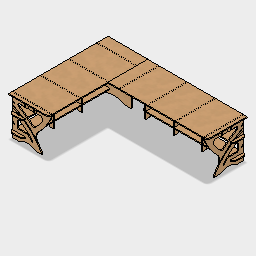
Corner bench (Autodesk Fusion 360 design; units mm, degrees)
Autodesk Fusion 360 part; units mm, degrees
note: some values were not read from the file. Set by a fixed rule: which sketch regions a step uses.
(part 1 of 2)
sketch "Inner end leg" plane through (0, 0, 0) normal (0, 0, 1) x (1, 0, 0)
  circle A0 centre (-454.5584, 695.833) radius 3.175
  line L0 (-307.4416, 743.458) -> (-289.4584, 743.458) construction
  line L1 (-454.5584, 692.658) -> (-472.5416, 692.658)
  line L2 (-472.5416, 692.658) -> (-472.5416, 749.6387)
  line L3 (-307.4416, 692.658) -> (-307.4416, 749.6387)
  circle A1 centre (-123.825, 133.858) radius 3.175
  line L4 (-454.5584, 749.6387) -> (-454.5584, 692.658)
  circle A2 centre (-307.4416, 695.833) radius 3.175
  circle A3 centre (-123.825, 115.8748) radius 3.175
  line L5 (-472.5416, 743.458) -> (-454.5584, 743.458) construction
  circle A4 centre (-472.5416, 695.833) radius 3.175
  circle A5 centre (-289.4584, 695.833) radius 3.175
  line L6 (-289.4584, 749.6387) -> (-289.4584, 692.658)
  line L7 (-289.4584, 692.658) -> (-307.4416, 692.658)
  line L8 (0, 288.3803) -> (-40.4112, 247.9691)
  line L9 (-31.4309, 238.9888) -> (-5.4201, 264.9997)
  arc A6 (-40.4112, 584.3498) -> (-31.4309, 575.3695) centre (-35.921, 579.8596) ccw
  arc A7 (-40.4112, 247.9691) -> (-31.4309, 238.9888) centre (-35.921, 243.479) ccw
  line L10 (0, 133.858) -> (-127, 133.858)
  line L11 (0, 429.6664) -> (-127, 429.6664) construction
  line L12 (-127, 115.8748) -> (0, 115.8748)
  line L13 (0, 124.8664) -> (-127, 124.8664) construction
  circle A8 centre (-123.825, 420.6748) radius 3.175
  line L14 (-127, 133.858) -> (-127, 115.8748)
  circle A9 centre (-123.825, 438.658) radius 3.175
  line L15 (0, 624.7609) -> (-40.4112, 584.3498)
  line L16 (-35.921, 579.8596) -> (0, 615.7807) construction
  line L17 (0, 438.658) -> (-127, 438.658)
  line L18 (0, 279.4) -> (-35.921, 243.479) construction
  line L19 (-31.4309, 575.3695) -> (-5.4201, 601.3803)
  line L20 (-127, 420.6748) -> (0, 420.6748)
  line L21 (-127, 438.658) -> (-127, 420.6748)
  line L22 (-660.4, 749.6387) -> (-660.4, 0)
  line L23 (-112.121, 629.158) -> (-558.8, 629.158)
  line L24 (-584.2, 603.758) -> (-584.2, 527.558)
  line L25 (-558.8, 502.158) -> (-112.121, 502.158)
  line L26 (-86.721, 527.558) -> (-86.721, 603.758)
  line L27 (-112.121, 357.1748) -> (-558.8, 357.1748)
  line L28 (-584.2, 331.7748) -> (-584.2, 222.758)
  line L29 (-558.8, 197.358) -> (-112.121, 197.358)
  line L30 (-86.721, 222.758) -> (-86.721, 331.7748)
  arc A10 (-86.721, 603.758) -> (-112.121, 629.158) centre (-112.121, 603.758) ccw
  arc A11 (-558.8, 629.158) -> (-584.2, 603.758) centre (-558.8, 603.758) ccw
  arc A12 (-584.2, 527.558) -> (-558.8, 502.158) centre (-558.8, 527.558) ccw
  arc A13 (-112.121, 502.158) -> (-86.721, 527.558) centre (-112.121, 527.558) ccw
  arc A14 (-86.721, 331.7748) -> (-112.121, 357.1748) centre (-112.121, 331.7748) ccw
  arc A15 (-558.8, 357.1748) -> (-584.2, 331.7748) centre (-558.8, 331.7748) ccw
  arc A16 (-584.2, 222.758) -> (-558.8, 197.358) centre (-558.8, 222.758) ccw
  arc A17 (-112.121, 197.358) -> (-86.721, 222.758) centre (-112.121, 222.758) ccw
  arc A18 (-101.6, 0) -> (-558.8, 0) centre (-330.2, -488.95) ccw
  line L31 (-660.4, 0) -> (-558.8, 0)
  line L32 (-101.6, 0) -> (0, 0)
  line L33 (0, 749.6387) -> (-289.4584, 749.6387)
  line L34 (-307.4416, 749.6387) -> (-454.5584, 749.6387)
  line L35 (-472.5416, 749.6387) -> (-660.4, 749.6387)
  line L36 (0, 624.7609) -> (0, 749.6387)
  line L37 (0, 599.1353) -> (0, 624.7609) construction
  line L38 (0, 438.658) -> (0, 599.1353)
  line L39 (0, 288.3803) -> (0, 420.6748)
  line L40 (0, 0) -> (0, 115.8748)
  line L41 (0, 400.0363) -> (0, 288.3803) construction
  line L42 (0, 133.858) -> (0, 262.7546)
  arc A19 (0, 599.1353) -> (-5.4201, 601.3803) centre (-3.175, 599.1353) ccw
  arc A20 (0, 262.7546) -> (-5.4201, 264.9997) centre (-3.175, 262.7546) ccw
  line L43 (0, 420.6748) -> (0, 438.658) construction
  line L44 (0, 115.8748) -> (0, 133.858) construction
  line L45 (0, 288.3803) -> (0, 262.7546) construction
  line L46 (-101.6, 0) -> (-558.8, 0) construction
  line L47 (-330.2, 0) -> (-330.2, 50.8) construction
  point P0 (0, 429.6664)
  point P1 (-298.45, 743.458)
  point P2 (-381, 749.6387)
  point P3 (-463.55, 743.458)
  point P4 (-558.8, 0)
  point P5 (-101.6, 0)
  dimension "d1011" = 50.8
  dimension "d1015" = 50.8
  dimension "d1017" = 17.9832
  dimension "d1019" = 6.35
  dimension "d1020" = 6.35
  dimension "d1021" = 17.9832
  dimension "d1023" = 6.35
  dimension "d1024" = 6.35
  dimension "d1025" = 8.9916
  dimension "d1026" = 8.9916
  dimension "d1034" = 50.8
  dimension "d1036" = 50.8
  dimension "d1037" = 6.35
  dimension "d1038" = 6.35
  dimension "d1039" = 6.35
  dimension "d1040" = 6.35
  dimension "d1042" = 82.55
  dimension "d1043" = 82.55
  dimension "d1062" = 133.858
  dimension "d1063" = 438.658
  dimension "d1103" = 63.5
  dimension "d1104" = 63.5
  dimension "d1105" = 50.8
  dimension "d1106" = 76.2
  dimension "d1107" = 76.2
  dimension "d1108" = 50.8
  dimension "d1109" = 63.5
  dimension "d1110" = 63.5
  dimension "d1114" = 25.4
  dimension "d1115" = 25.4
  dimension "d1250" = 101.6
  dimension "d2612" = 3.175
  dimension "d2613" = 3.175
  dimension "d2750" = 6.35
  dimension "d2751" = 6.35
  dimension "d2961" = 45
  dimension "d2962" = 127
  dimension "d2964" = 101.6
  dimension "d2965" = 127
  dimension "d2966" = 45
  dimension "d2967" = 279.4
  dimension "d2969" = 6.1807
  dimension "d2970" = 6.1807
  dimension "d2971" = 660.4
  dimension "d2972" = 749.6387
  dimension "d2973" = 279.4
  dimension "d2974" = 17.9832
  dimension "d2975" = 17.9832
  dimension "d2976" = 133.858
  dimension "d3349" = 50.8
  measures "d1011" distance of A6.centre L16.end
  measures "d1015" distance of L18.start A7.centre
  measures "d1017" distance of L17 L20
  measures "d1019" diameter of A8
  measures "d1020" diameter of A9
  measures "d1021" distance of L10 L12
  measures "d1023" diameter of A3
  measures "d1024" diameter of A1
  measures "d1025" distance of L11 L20
  measures "d1026" distance of L12 L13
  measures "d1034" distance of L1.end L5.start
  measures "d1036" distance of L3.start L0.start
  measures "d1037" diameter of A0
  measures "d1038" diameter of A4
  measures "d1039" diameter of A5
  measures "d1040" diameter of A2
  measures "d1042" distance of P2 P3
  measures "d1043" distance of P1 P2
  measures "d1062" distance of L32.end L10
  measures "d1063" distance of L32.end L17
  measures "d1103" distance of L7 L23
  measures "d1104" distance of L17 L25
  measures "d1105" distance of A6.centre L26
  measures "d1106" distance of L22 L24
  measures "d1107" distance of L22 L28
  measures "d1108" distance of A7.centre L30
  measures "d1109" distance of L20 L27
  measures "d1110" distance of L10 L29
  measures "d1114" radius of A10
  measures "d1115" radius of A14
  measures "d1250" distance of P5 L32.end
  measures "d2612" radius of A19
  measures "d2613" radius of A20
  measures "d2750" radius of A6
  measures "d2751" radius of A7
  measures "d2961" angle of L16 L38
  measures "d2962" distance of L21 L43
  measures "d2964" distance of L22.end P4
  measures "d2965" distance of L14 L44
  measures "d2966" angle of L18 L42
  measures "d2967" distance of L32.end L18.start
  measures "d2969" distance of L0 L34
  measures "d2970" distance of L5 L34
  measures "d2971" distance of L22 L36
  measures "d2972" distance of L31 L35
  measures "d2973" distance of P2 L22
  measures "d2974" distance of L2 L4
  measures "d2975" distance of L3 L6
  measures "d2976" distance of L16.end L33
  measures "d3349" distance of L47.start L47.end
sketch "End leg - wave" plane through (0, 0, 0) normal (1, 0, 0) x (0, 0, -1)
  arc A0 (0, 0) -> (-89.7433, 139.7) centre (-1260.9786, -711.3774) ccw
  arc A1 (-74.171, 337.0976) -> (190.5, 744.1354) centre (-899.991, 1163.6445) ccw
  arc A2 (-127, 0) -> (-444.5, 0) centre (-285.75, -222.6469) ccw
  line L0 (0, 0) -> (-127, 0)
  line L1 (-444.5, 0) -> (-571.5, 0)
  arc A3 (-113.8369, 190.5) -> (-571.5, 547.1161) centre (-1134.6675, -647.6035) ccw
  line L2 (-571.5, 438.658) -> (-444.5, 438.658)
  line L3 (-444.5, 438.658) -> (-444.5, 420.6748)
  line L4 (-444.5, 420.6748) -> (-450.85, 420.6748)
  circle A4 centre (-447.675, 438.658) radius 3.175
  line L5 (-571.5, 133.858) -> (-444.5, 133.858)
  line L6 (-444.5, 133.858) -> (-444.5, 115.8748)
  line L7 (-444.5, 115.8748) -> (-571.5, 115.8748)
  circle A5 centre (-447.675, 133.858) radius 3.175
  circle A6 centre (-447.675, 115.8748) radius 3.175
  arc A7 (-540.0691, 238.9888) -> (-531.0888, 247.9691) centre (-535.579, 243.479) ccw
  line L8 (-531.0888, 247.9691) -> (-571.5, 288.3803)
  line L9 (-571.5, 279.4) -> (-535.579, 243.479) construction
  arc A8 (-540.0691, 582.9049) -> (-531.0888, 591.8852) centre (-535.579, 587.3951) ccw
  line L10 (-531.0888, 591.8852) -> (-571.5, 632.2964)
  line L11 (-571.5, 623.3161) -> (-535.579, 587.3951) construction
  line L12 (-566.0799, 608.9158) -> (-540.0691, 582.9049)
  line L13 (-566.0799, 264.9997) -> (-540.0691, 238.9888)
  line L14 (-98.9584, 743.331) -> (-116.9416, 743.331) construction
  line L15 (-116.9416, 698.881) -> (-116.9416, 692.531)
  line L16 (-116.9416, 692.531) -> (-98.9584, 692.531)
  line L17 (-98.9584, 692.531) -> (-98.9584, 698.881)
  line L18 (-264.0584, 744.0968) -> (-282.0416, 744.0968) construction
  line L19 (-282.0416, 699.6468) -> (-282.0416, 693.2968)
  line L20 (-282.0416, 693.2968) -> (-264.0584, 693.2968)
  line L21 (-264.0584, 693.2968) -> (-264.0584, 699.6468)
  arc A9 (-74.171, 337.0976) -> (-89.7433, 139.7) centre (33.5446, 229.2871) ccw
  line L22 (-571.5, 438.658) -> (-571.5, 606.6707)
  line L23 (-571.5, 632.2964) -> (-571.5, 750.3161)
  line L24 (-98.9584, 698.881) -> (-98.9584, 743.331)
  line L25 (-116.9416, 743.331) -> (-116.9416, 698.881)
  line L26 (-264.0584, 699.6468) -> (-264.0584, 744.0968)
  line L27 (-282.0416, 744.0968) -> (-282.0416, 699.6468)
  arc A10 (-98.9584, 698.881) -> (-98.9584, 692.531) centre (-98.9584, 695.706) ccw
  arc A11 (-98.9584, 692.531) -> (-98.9584, 698.881) centre (-98.9584, 695.706) ccw
  arc A12 (-116.9416, 692.531) -> (-116.9416, 698.881) centre (-116.9416, 695.706) ccw
  arc A13 (-116.9416, 698.881) -> (-116.9416, 692.531) centre (-116.9416, 695.706) ccw
  arc A14 (-264.0584, 699.6468) -> (-264.0584, 693.2968) centre (-264.0584, 696.4718) ccw
  arc A15 (-264.0584, 693.2968) -> (-264.0584, 699.6468) centre (-264.0584, 696.4718) ccw
  arc A16 (-282.0416, 693.2968) -> (-282.0416, 699.6468) centre (-282.0416, 696.4718) ccw
  arc A17 (-282.0416, 699.6468) -> (-282.0416, 693.2968) centre (-282.0416, 696.4718) ccw
  line L28 (-438.1501, 629.031) -> (-38.71, 629.031)
  arc A18 (-128.0289, 391.0028) -> (3.3037, 549.6743) centre (-899.991, 1163.6445) ccw
  line L29 (-463.5501, 603.631) -> (-463.5501, 607.3706)
  arc A19 (-128.0289, 391.0028) -> (-128.1972, 390.8344) centre (33.5446, 229.2871) ccw
  arc A20 (-198.1934, 389.0378) -> (-438.0805, 563.3364) centre (-1134.6675, -647.6035) ccw
  arc A21 (-89.7433, 139.7) -> (-571.5, 496.3161) centre (-896.6375, -446.6291) ccw
  arc A22 (-444.5, 420.6748) -> (-450.85, 420.6748) centre (-447.675, 420.6748) ccw
  arc A23 (-450.85, 420.6748) -> (-444.5, 420.6748) centre (-447.675, 420.6748) ccw
  line L30 (-450.85, 420.6748) -> (-571.5, 420.6748)
  arc A24 (-182.2534, 135.0186) -> (-433.921, 349.9587) centre (-896.6375, -446.6291) ccw
  line L31 (-472.079, 327.9952) -> (-472.079, 222.758)
  arc A25 (3.3037, 549.6743) -> (-38.71, 629.031) centre (-38.71, 578.231) ccw
  arc A26 (-198.1934, 389.0378) -> (-128.1972, 390.8344) centre (-164.1398, 426.7338) ccw
  arc A27 (-463.5501, 607.3706) -> (-438.0805, 563.3364) centre (-412.7501, 607.3706) ccw
  arc A28 (-438.1501, 629.031) -> (-463.5501, 603.631) centre (-438.1501, 603.631) ccw
  arc A29 (-433.921, 349.9587) -> (-472.079, 327.9952) centre (-446.679, 327.9952) ccw
  line L32 (-294.8076, 197.358) -> (-446.679, 197.358)
  arc A30 (-201.9503, 118.9814) -> (-182.2534, 135.0186) centre (-192.1019, 127) ccw
  arc A31 (-472.079, 222.758) -> (-446.679, 197.358) centre (-446.679, 222.758) ccw
  line L33 (190.5, 744.1354) -> (190.5, 750.3161)
  line L34 (190.5, 750.3161) -> (-98.8844, 750.3161)
  line L35 (-98.8844, 750.3161) -> (-98.9584, 743.331)
  line L36 (-116.9416, 743.331) -> (-116.9416, 750.3161)
  line L37 (-116.9416, 750.3161) -> (-263.9925, 750.3161)
  line L38 (-263.9925, 750.3161) -> (-264.0584, 744.0968)
  line L39 (-282.0416, 744.0968) -> (-282.0416, 750.3161)
  line L40 (-282.0416, 750.3161) -> (-571.5, 750.3161)
  line L41 (-571.5, 288.3803) -> (-571.5, 420.6748)
  line L42 (-571.5, 0) -> (-571.5, 115.8748)
  line L43 (-571.5, 133.858) -> (-571.5, 262.7546)
  arc A32 (-566.0799, 264.9997) -> (-571.5, 262.7546) centre (-568.325, 262.7546) ccw
  line L44 (-571.5, 632.2964) -> (-571.5, 606.6707) construction
  arc A33 (-566.0799, 608.9158) -> (-571.5, 606.6707) centre (-568.325, 606.6707) ccw
  line L45 (-571.5, 288.3803) -> (-571.5, 262.7546) construction
  arc A34 (-201.9503, 118.9814) -> (-258.6277, 182.2183) centre (-896.6375, -446.6291) ccw
  arc A35 (-258.6277, 182.2183) -> (-294.8076, 197.358) centre (-294.8076, 146.558) ccw
  line L46 (-127, 0) -> (-444.5, 0) construction
  line L47 (-285.75, 0) -> (-285.75, 50.8) construction
  point P0 (-107.95, 743.331)
  point P1 (-273.05, 744.0968)
  point P2 (-190.5, 750.3161)
  dimension "d27" = 571.5
  dimension "d37" = 127
  dimension "d38" = 127
  dimension "d328" = 127
  dimension "d329" = 6.35
  dimension "d330" = 6.35
  dimension "d331" = 17.9832
  dimension "d332" = 438.658
  dimension "d333" = 127
  dimension "d334" = 17.9832
  dimension "d335" = 6.35
  dimension "d336" = 6.35
  dimension "d337" = 133.858
  dimension "d382" = 12.7
  dimension "d383" = 279.4
  dimension "d384" = 50.8
  dimension "d385" = 12.7
  dimension "d386" = 50.8
  dimension "d869" = 17.9832
  dimension "d870" = 50.8
  dimension "d871" = 17.9832
  dimension "d872" = 50.8
  dimension "d876" = 82.55
  dimension "d877" = 82.55
  dimension "d878" = 6.35
  dimension "d879" = 6.35
  dimension "d880" = 6.35
  dimension "d881" = 6.35
  dimension "d1120" = 63.5
  dimension "d1122" = 76.2
  dimension "d1127" = 76.2
  dimension "d1130" = 63.5
  dimension "d1131" = 50.8
  dimension "d1132" = 50.8
  dimension "d1133" = 50.8
  dimension "d1134" = 25.4
  dimension "d1136" = 25.4
  dimension "d1143" = 63.5
  dimension "d1148" = 25.4
  dimension "d2090" = 997.4268
  dimension "d2570" = 3.175
  dimension "d2578" = 107.95
  dimension "d2579" = 127
  dimension "d2580" = 3.175
  dimension "d2978" = 45
  dimension "d2979" = 381
  dimension "d2980" = 6.1807
  dimension "d2981" = 762
  dimension "d2982" = 203.2
  dimension "d2985" = 50.8
  dimension "d2987" = 750.3161
  dimension "d2989" = 1168.4
  dimension "d2990" = 152.4
  dimension "d2991" = 1447.8
  dimension "d2993" = 45
  dimension "d2994" = 139.7
  dimension "d2995" = 50.8
  dimension "d2999" = 12.7
  dimension "d3001" = 50.8
  dimension "d3002" = 127
  dimension "d3003" = 76.2
  dimension "d3004" = 1320.8
  dimension "d3350" = 50.8
  measures "d27" distance of A0.start L1.end
  measures "d37" distance of A0.start A2.start
  measures "d38" distance of L1.end A2.end
  measures "d328" distance of L2.start L2.end
  measures "d329" diameter of A22
  measures "d330" diameter of A4
  measures "d331" distance of L2 L4
  measures "d332" distance of L1 L2
  measures "d333" distance of L5.start L5.end
  measures "d334" distance of L5.start L7.end
  measures "d335" diameter of A5
  measures "d336" diameter of A6
  measures "d337" distance of L1 L5
  measures "d382" diameter of A7
  measures "d383" distance of L1 L9.start
  measures "d384" distance of L9.start A7.centre
  measures "d385" diameter of A8
  measures "d386" distance of L11.start A8.centre
  measures "d869" distance of L14.start L14.end
  measures "d870" distance of L14.start L16.end
  measures "d871" distance of L18.start L18.end
  measures "d872" distance of L18.start L20.end
  measures "d876" distance of P0 P2
  measures "d877" distance of P1 P2
  measures "d878" diameter of A12
  measures "d879" diameter of A10
  measures "d880" diameter of A14
  measures "d881" diameter of A16
  measures "d1120" distance of L16 L28
  measures "d1122" distance of A1 A18
  measures "d1127" distance of A21 A24
  measures "d1130" distance of A7.centre L31
  measures "d1131" radius of A25
  measures "d1132" radius of A26
  measures "d1133" radius of A27
  measures "d1134" radius of A28
  measures "d1136" radius of A29
  measures "d1143" distance of L5 L32
  measures "d1148" radius of A31
  measures "d2090" radius of A21
  measures "d2570" radius of A32
  measures "d2578" distance of L23 L29
  measures "d2579" distance of L11.start L40
  measures "d2580" radius of A33
  measures "d2978" angle of L11 L22
  measures "d2979" distance of P2 L23
  measures "d2980" distance of A1.end L33.end
  measures "d2981" distance of L23 L33
  measures "d2982" distance of A3.end L23.end
  measures "d2985" distance of A3.end A21.end
  measures "d2987" distance of L1 L40
  measures "d2989" radius of A1
  measures "d2990" radius of A9
  measures "d2991" radius of A0
  measures "d2993" angle of L9 L43
  measures "d2994" distance of L0 A0.end
  measures "d2995" distance of A3.start A0.end
  measures "d2999" radius of A30
  measures "d3001" radius of A35
  measures "d3002" distance of A0.start A30.centre
  measures "d3003" distance of A3 A20
  measures "d3004" radius of A3
  measures "d3350" distance of L47.start L47.end
sketch "Spine - short" plane through (0, 0, 0) normal (1, 0, 0) x (0, 0, -1)
  line L0 (1828.8, 50.8) -> (1828.8, 101.6)
  line L1 (0, 101.6) -> (0, 50.8)
  line L2 (1774.2916, 0) -> (1756.3084, 0) construction
  line L3 (1756.3084, 0) -> (1756.3084, 50.8)
  line L4 (1756.3084, 50.8) -> (1774.2916, 50.8)
  line L5 (1774.2916, 50.8) -> (1774.2916, 0)
  line L6 (1216.5584, 0) -> (1216.5584, 50.8)
  line L7 (1216.5584, 50.8) -> (1234.5416, 50.8)
  line L8 (1234.5416, 50.8) -> (1234.5416, 0)
  line L9 (694.7916, 0) -> (676.8084, 0) construction
  line L10 (676.8084, 0) -> (676.8084, 50.8)
  line L11 (676.8084, 50.8) -> (694.7916, 50.8)
  line L12 (694.7916, 50.8) -> (694.7916, 0)
  line L13 (155.0416, 0) -> (137.0584, 0) construction
  line L14 (137.0584, 0) -> (137.0584, 50.8)
  line L15 (137.0584, 50.8) -> (155.0416, 50.8)
  line L16 (155.0416, 50.8) -> (155.0416, 0)
  circle A0 centre (1756.3084, 47.625) radius 3.175
  circle A1 centre (1774.2916, 47.625) radius 3.175
  circle A2 centre (1234.5416, 47.625) radius 3.175
  circle A3 centre (1216.5584, 47.625) radius 3.175
  circle A4 centre (694.7916, 47.625) radius 3.175
  circle A5 centre (676.8084, 47.625) radius 3.175
  circle A6 centre (155.0416, 47.625) radius 3.175
  circle A7 centre (137.0584, 47.625) radius 3.175
  line L17 (247.3706, 101.6) -> (247.3706, 50.8)
  line L18 (247.3706, 50.8) -> (229.3874, 50.8)
  line L19 (229.3874, 50.8) -> (229.3874, 101.6)
  line L20 (412.4706, 101.6) -> (412.4706, 50.8)
  line L21 (412.4706, 50.8) -> (394.4874, 50.8)
  line L22 (394.4874, 50.8) -> (394.4874, 101.6)
  circle A8 centre (229.3874, 53.975) radius 3.175
  circle A9 centre (247.3706, 53.975) radius 3.175
  circle A10 centre (394.4874, 53.975) radius 3.175
  circle A11 centre (412.4706, 53.975) radius 3.175
  arc A12 (1778, 0) -> (1828.8, 50.8) centre (1778, 50.8) ccw
  arc A13 (0, 50.8) -> (50.8, 0) centre (50.8, 50.8) ccw
  line L23 (1774.2916, 0) -> (1778, 0)
  line L24 (1234.5416, 0) -> (1756.3084, 0)
  line L25 (1216.5584, 0) -> (1234.5416, 0) construction
  line L26 (694.7916, 0) -> (1216.5584, 0)
  line L27 (1828.8, 101.6) -> (412.4706, 101.6)
  line L28 (412.4706, 101.6) -> (394.4874, 101.6) construction
  line L29 (394.4874, 101.6) -> (247.3706, 101.6)
  line L30 (229.3874, 101.6) -> (0, 101.6)
  line L31 (247.3706, 101.6) -> (229.3874, 101.6) construction
  line L32 (50.8, 0) -> (137.0584, 0)
  line L33 (155.0416, 0) -> (676.8084, 0)
  point P0 (1828.8, 0)
  point P1 (146.05, 0)
  point P2 (685.8, 0)
  point P3 (1225.55, 0)
  point P4 (1765.3, 0)
  point P5 (238.379, 101.6)
  point P6 (403.479, 101.6)
  dimension "d906" = 1828.8
  dimension "d907" = 101.6
  dimension "d908" = 17.9832
  dimension "d909" = 50.8
  dimension "d912" = 17.9832
  dimension "d913" = 50.8
  dimension "d914" = 17.9832
  dimension "d915" = 50.8
  dimension "d916" = 17.9832
  dimension "d917" = 50.8
  dimension "d921" = 539.75
  dimension "d922" = 539.75
  dimension "d924" = 63.5
  dimension "d925" = 539.75
  dimension "d928" = 6.35
  dimension "d929" = 6.35
  dimension "d930" = 6.35
  dimension "d931" = 6.35
  dimension "d932" = 6.35
  dimension "d933" = 6.35
  dimension "d934" = 6.35
  dimension "d935" = 6.35
  dimension "d948" = 120.65
  dimension "d969" = 17.9832
  dimension "d970" = 50.8
  dimension "d972" = 50.8
  dimension "d973" = 6.35
  dimension "d974" = 6.35
  dimension "d975" = 6.35
  dimension "d976" = 6.35
  dimension "d977" = 92.329
  dimension "d978" = 165.1
  dimension "d982" = 50.8
  dimension "d983" = 50.8
  dimension "d1382" = 17.9832
  measures "d906" distance of origin P0
  measures "d907" distance of origin L1.start
  measures "d908" distance of L2.start L2.end
  measures "d909" distance of L2.start L4.end
  measures "d912" distance of L8.end L6.start
  measures "d913" distance of L7.end L8.end
  measures "d914" distance of L9.start L9.end
  measures "d915" distance of L11.end L9.start
  measures "d916" distance of L13.start L13.end
  measures "d917" distance of L15.end L13.start
  measures "d921" distance of P2 P3
  measures "d922" distance of P1 P2
  measures "d924" distance of L0 P4
  measures "d925" distance of P3 P4
  measures "d928" diameter of A1
  measures "d929" diameter of A0
  measures "d930" diameter of A2
  measures "d931" diameter of A3
  measures "d932" diameter of A4
  measures "d933" diameter of A5
  measures "d934" diameter of A6
  measures "d935" diameter of A7
  measures "d969" distance of L19.end L17.start
  measures "d970" distance of L19.end L18.end
  measures "d972" distance of L22.end L21.end
  measures "d973" diameter of A11
  measures "d974" diameter of A10
  measures "d975" diameter of A9
  measures "d976" diameter of A8
  measures "d977" distance of P1 P5
  measures "d978" distance of P5 P6
  measures "d982" radius of A12
  measures "d983" radius of A13
  measures "d1382" distance of L20 L22
sketch "Shelf" plane through (0, 0, 0) normal (0, 1, 0) x (1, 0, 0)
  line L0 (50.8, 0) -> (203.2, 0)
  line L1 (254, 50.8) -> (254, 1695.45)
  line L2 (203.2, 1746.25) -> (50.8, 1746.25)
  line L3 (0, 1673.7584) -> (127, 1673.7584)
  line L4 (127, 1673.7584) -> (127, 1691.7416)
  line L5 (127, 1691.7416) -> (0, 1691.7416)
  arc A0 (50.8, 1746.25) -> (0, 1695.45) centre (50.8, 1695.45) ccw
  arc A1 (254, 1695.45) -> (203.2, 1746.25) centre (203.2, 1695.45) ccw
  arc A2 (0, 50.8) -> (50.8, 0) centre (50.8, 50.8) ccw
  arc A3 (203.2, 0) -> (254, 50.8) centre (203.2, 50.8) ccw
  line L6 (0, 0) -> (0, 20.32) construction
  line L7 (0, 0) -> (20.32, 0) construction
  line L8 (0, 1134.0084) -> (127, 1134.0084)
  line L9 (127, 1134.0084) -> (127, 1151.9916)
  line L10 (127, 1151.9916) -> (0, 1151.9916)
  line L11 (0, 1151.9916) -> (0, 1134.0084) construction
  line L12 (0, 594.2584) -> (127, 594.2584)
  line L13 (127, 594.2584) -> (127, 612.2416)
  line L14 (127, 612.2416) -> (0, 612.2416)
  line L15 (0, 72.4916) -> (127, 72.4916)
  line L16 (127, 72.4916) -> (127, 54.5084)
  line L17 (127, 54.5084) -> (0, 54.5084)
  circle A4 centre (123.825, 54.5084) radius 3.175
  circle A5 centre (123.825, 72.4916) radius 3.175
  circle A6 centre (123.825, 594.2584) radius 3.175
  circle A7 centre (123.825, 612.2416) radius 3.175
  circle A8 centre (123.825, 1134.0084) radius 3.175
  circle A9 centre (123.825, 1151.9916) radius 3.175
  circle A10 centre (123.825, 1691.7416) radius 3.175
  circle A11 centre (123.825, 1673.7584) radius 3.175
  line L18 (0, 1695.45) -> (0, 1691.7416)
  line L19 (0, 1673.7584) -> (0, 1151.9916)
  line L20 (0, 1134.0084) -> (0, 612.2416)
  line L21 (0, 612.2416) -> (0, 594.2584) construction
  line L22 (0, 594.2584) -> (0, 72.4916)
  line L23 (0, 54.5084) -> (0, 50.8)
  line L24 (0, 72.4916) -> (0, 54.5084) construction
  line L25 (0, 1691.7416) -> (0, 1673.7584) construction
  point P0 (0, 1682.75)
  point P1 (0, 1143)
  point P2 (0, 603.25)
  point P3 (0, 63.5)
  dimension "d493" = 127
  dimension "d494" = 17.9832
  dimension "d496" = 50.8
  dimension "d497" = 50.8
  dimension "d498" = 50.8
  dimension "d499" = 50.8
  dimension "d500" = 127
  dimension "d501" = 17.9832
  dimension "d502" = 539.75
  dimension "d503" = 17.9832
  dimension "d504" = 127
  dimension "d505" = 539.75
  dimension "d506" = 127
  dimension "d507" = 17.9832
  dimension "d508" = 539.75
  dimension "d509" = 6.35
  dimension "d510" = 6.35
  dimension "d511" = 6.35
  dimension "d512" = 6.35
  dimension "d513" = 6.35
  dimension "d514" = 6.35
  dimension "d515" = 6.35
  dimension "d516" = 6.35
  dimension "d980" = 63.5
  dimension "d3017" = 254
  dimension "d3592" = 63.5
  dimension "d3593" = 1746.25
  measures "d493" distance of L3.start L3.end
  measures "d494" distance of L3.start L5.end
  measures "d496" radius of A0
  measures "d497" radius of A1
  measures "d498" radius of A2
  measures "d499" radius of A3
  measures "d500" distance of L8.start L8.end
  measures "d501" distance of L8.start L10.end
  measures "d502" distance of P0 P1
  measures "d503" distance of L12.start L14.end
  measures "d504" distance of L12.start L12.end
  measures "d505" distance of P1 P2
  measures "d506" distance of L15.start L15.end
  measures "d507" distance of L15.start L17.end
  measures "d508" distance of P2 P3
  measures "d509" diameter of A5
  measures "d510" diameter of A4
  measures "d511" diameter of A7
  measures "d512" diameter of A6
  measures "d513" diameter of A9
  measures "d514" diameter of A8
  measures "d515" diameter of A10
  measures "d516" diameter of A11
  measures "d980" distance of L2 P0
  measures "d3017" distance of L1 L20
  measures "d3592" distance of L0 P3
  measures "d3593" distance of L0 L2
sketch "Inner leg" plane through (0, 0, 0) normal (0, 0, 1) x (1, 0, 0)
  line L0 (-660.4, 749.6387) -> (-660.4, 686.1387)
  line L1 (-254, 0) -> (-254, 305.1387)
  line L2 (-584.2, 609.9387) -> (-558.8, 609.9387)
  arc A0 (-660.4, 686.1387) -> (-584.2, 609.9387) centre (-584.2, 686.1387) ccw
  arc A1 (-254, 305.1387) -> (-558.8, 609.9387) centre (-558.8, 305.1387) ccw
  line L3 (0, 622.6387) -> (-35.921, 586.7176) construction
  line L4 (-31.4309, 582.2275) -> (-5.4201, 608.2383)
  line L5 (0, 631.6189) -> (-40.4112, 591.2078)
  arc A2 (-40.4112, 591.2078) -> (-31.4309, 582.2275) centre (-35.921, 586.7176) ccw
  line L6 (0, 288.3803) -> (-40.4112, 247.9691)
  arc A3 (-40.4112, 247.9691) -> (-31.4309, 238.9888) centre (-35.921, 243.479) ccw
  line L7 (-31.4309, 238.9888) -> (-5.4201, 264.9997)
  line L8 (0, 279.4) -> (-35.921, 243.479) construction
  line L9 (0, 438.658) -> (-127, 438.658)
  line L10 (-127, 420.6748) -> (0, 420.6748)
  line L11 (0, 429.6664) -> (-127, 429.6664) construction
  line L12 (-127, 438.658) -> (-127, 420.6748)
  circle A4 centre (-123.825, 438.658) radius 3.175
  circle A5 centre (-123.825, 420.6748) radius 3.175
  line L13 (0, 133.858) -> (-127, 133.858)
  line L14 (-127, 115.8748) -> (0, 115.8748)
  line L15 (0, 123.0376) -> (-127, 123.0376) construction
  line L16 (-127, 133.858) -> (-127, 115.8748)
  circle A6 centre (-123.825, 133.858) radius 3.175
  circle A7 centre (-123.825, 115.8748) radius 3.175
  line L17 (-472.6264, 743.458) -> (-454.6432, 743.458) construction
  line L18 (-454.6432, 749.6387) -> (-454.6432, 692.658)
  line L19 (-454.6432, 692.658) -> (-472.6264, 692.658)
  line L20 (-472.6264, 692.658) -> (-472.6264, 749.6387)
  line L21 (-307.5264, 743.458) -> (-289.5432, 743.458) construction
  line L22 (-289.5432, 749.6387) -> (-289.5432, 692.658)
  line L23 (-289.5432, 692.658) -> (-307.5264, 692.658)
  line L24 (-307.5264, 692.658) -> (-307.5264, 749.6387)
  circle A8 centre (-472.6264, 695.833) radius 3.175
  circle A9 centre (-454.6432, 695.833) radius 3.175
  circle A10 centre (-307.5264, 695.833) radius 3.175
  circle A11 centre (-289.5432, 695.833) radius 3.175
  line L25 (-264.1432, 603.758) -> (-304.598, 603.758)
  line L26 (-196.6258, 489.458) -> (-114.3, 489.458)
  arc A12 (-239.2345, 512.5969) -> (-308.7652, 592.6167) centre (-558.8, 305.1387) ccw
  line L27 (-88.9, 514.858) -> (-88.9, 641.6887)
  line L28 (-114.3, 667.0887) -> (-213.3432, 667.0887)
  line L29 (-238.7432, 641.6887) -> (-238.7432, 629.158)
  arc A13 (-88.9, 641.6887) -> (-114.3, 667.0887) centre (-114.3, 641.6887) ccw
  arc A14 (-114.3, 489.458) -> (-88.9, 514.858) centre (-114.3, 514.858) ccw
  arc A15 (-213.3432, 667.0887) -> (-238.7432, 641.6887) centre (-213.3432, 641.6887) ccw
  arc A16 (-264.1432, 603.758) -> (-238.7432, 629.158) centre (-264.1432, 629.158) ccw
  arc A17 (-304.598, 603.758) -> (-308.7652, 592.6167) centre (-304.598, 597.408) ccw
  arc A18 (-239.2345, 512.5969) -> (-196.6258, 489.458) centre (-196.6258, 540.258) ccw
  line L30 (-114.3, 357.1748) -> (-152.4, 357.1748)
  line L31 (-177.8, 331.7748) -> (-177.8, 222.758)
  line L32 (-152.4, 197.358) -> (-114.3, 197.358)
  line L33 (-88.9, 222.758) -> (-88.9, 331.7748)
  arc A19 (-152.4, 357.1748) -> (-177.8, 331.7748) centre (-152.4, 331.7748) ccw
  arc A20 (-88.9, 331.7748) -> (-114.3, 357.1748) centre (-114.3, 331.7748) ccw
  arc A21 (-177.8, 222.758) -> (-152.4, 197.358) centre (-152.4, 222.758) ccw
  arc A22 (-114.3, 197.358) -> (-88.9, 222.758) centre (-114.3, 222.758) ccw
  line L34 (-660.4, 749.6387) -> (-472.6264, 749.6387)
  line L35 (-454.6432, 749.6387) -> (-307.5264, 749.6387)
  line L36 (-289.5432, 749.6387) -> (0, 749.6387)
  line L37 (0, 631.6189) -> (0, 749.6387)
  line L38 (0, 438.658) -> (0, 605.9933)
  line L39 (0, 133.858) -> (0, 262.7546)
  line L40 (0, 288.3803) -> (0, 420.6748)
  line L41 (0, 631.6189) -> (0, 613.6584) construction
  arc A23 (0, 605.9933) -> (-5.4201, 608.2383) centre (-3.175, 605.9933) ccw
  line L42 (0, 288.3803) -> (0, 262.7546) construction
  arc A24 (0, 262.7546) -> (-5.4201, 264.9997) centre (-3.175, 262.7546) ccw
  line L43 (0, 0) -> (0, 115.8748)
  line L44 (0, 0) -> (-76.2, 0)
  line L45 (-177.8, 0) -> (-254, 0)
  line L46 (-76.2, 0) -> (-177.8, 0) construction
  line L47 (0, 133.858) -> (0, 115.8748) construction
  line L48 (0, 438.658) -> (0, 420.6748) construction
  arc A25 (-76.2, 0) -> (-177.8, 0) centre (-127, -38.1) ccw
  line L49 (-127, 0) -> (-127, 25.4) construction
  point P0 (-463.6348, 743.458)
  point P1 (-298.5348, 743.458)
  point P2 (-381.0848, 749.6387)
  point P3 (0, 429.6664)
  point P4 (0, 123.0376)
  point P5 (-127, 0)
  dimension "d103" = 254
  dimension "d110" = 76.2
  dimension "d113" = 304.8
  dimension "d262" = 50.8
  dimension "d304" = 50.8
  dimension "d314" = 17.9832
  dimension "d316" = 6.35
  dimension "d317" = 6.35
  dimension "d320" = 17.9832
  dimension "d322" = 6.35
  dimension "d323" = 6.35
  dimension "d772" = 17.9832
  dimension "d773" = 50.8
  dimension "d774" = 17.9832
  dimension "d775" = 50.8
  dimension "d776" = 6.35
  dimension "d777" = 6.35
  dimension "d778" = 6.35
  dimension "d779" = 6.35
  dimension "d782" = 82.55
  dimension "d783" = 82.55
  dimension "d1075" = 381
  dimension "d1083" = 50.8
  dimension "d1084" = 50.8
  dimension "d1085" = 25.4
  dimension "d1086" = 25.4
  dimension "d1087" = 25.4
  dimension "d1088" = 25.4
  dimension "d1089" = 6.35
  dimension "d1090" = 50.8
  dimension "d1092" = 63.5
  dimension "d1093" = 76.2
  dimension "d1094" = 63.5
  dimension "d1095" = 25.4
  dimension "d2571" = 88.9
  dimension "d2572" = 82.55
  dimension "d2573" = 3.175
  dimension "d2574" = 88.9
  dimension "d2575" = 3.175
  dimension "d2576" = 127
  dimension "d2577" = 88.9
  dimension "d3021" = 127
  dimension "d3022" = 127
  dimension "d3023" = 45
  dimension "d3024" = 749.6387
  dimension "d3025" = 133.858
  dimension "d3026" = 279.4
  dimension "d3027" = 438.658
  dimension "d3028" = 127
  dimension "d3029" = 45
  dimension "d3030" = 6.35
  dimension "d3031" = 139.7
  dimension "d3032" = 6.1807
  dimension "d3033" = 289.5432
  dimension "d3034" = 6.1807
  dimension "d3035" = 660.4
  dimension "d3036" = 6.35
  dimension "d3037" = 88.9
  dimension "d3375" = 25.4
  dimension "d3376" = 76.2
  measures "d103" distance of L43.start L1.start
  measures "d110" radius of A0
  measures "d113" radius of A1
  measures "d262" distance of L3.start L3.end
  measures "d304" distance of L8.start A3.centre
  measures "d314" distance of L9 L10
  measures "d316" diameter of A5
  measures "d317" diameter of A4
  measures "d320" distance of L13 L14
  measures "d322" diameter of A7
  measures "d323" diameter of A6
  measures "d772" distance of L17.start L17.end
  measures "d773" distance of L17.start L19.end
  measures "d774" distance of L21.start L21.end
  measures "d775" distance of L21.start L23.end
  measures "d776" diameter of A9
  measures "d777" diameter of A8
  measures "d778" diameter of A11
  measures "d779" diameter of A10
  measures "d782" distance of P0 P2
  measures "d783" distance of P1 P2
  measures "d1075" radius of A12
  measures "d1083" distance of L22 L29
  measures "d1084" distance of L9 L26
  measures "d1085" radius of A13
  measures "d1086" radius of A14
  measures "d1087" radius of A15
  measures "d1088" radius of A16
  measures "d1089" radius of A17
  measures "d1090" radius of A18
  measures "d1092" distance of L10 L30
  measures "d1093" distance of L1 L31
  measures "d1094" distance of L13 L32
  measures "d1095" radius of A19
  measures "d2571" distance of L27 L37
  measures "d2572" distance of L28 L36
  measures "d2573" radius of A23
  measures "d2574" distance of L33 L40
  measures "d2575" radius of A24
  measures "d2576" distance of L3.start L36
  measures "d2577" distance of L27 L38
  measures "d3021" distance of P5 L43.start
  measures "d3022" distance of L16 L47
  measures "d3023" angle of L8 L39
  measures "d3024" distance of L36 L44
  measures "d3025" distance of L13 L44
  measures "d3026" distance of L8.start L44
  measures "d3027" distance of L9 L44
  measures "d3028" distance of L12 L48
  measures "d3029" angle of L3 L38
  measures "d3030" radius of A2
  measures "d3031" distance of L2.start L34
  measures "d3032" distance of L21 L36
  measures "d3033" distance of L22 L37
  measures "d3034" distance of L17 L35
  measures "d3035" distance of L0 L37
  measures "d3036" radius of A3
  measures "d3037" distance of L23 L25
  measures "d3375" distance of P5 L49.end
  measures "d3376" distance of L44.end L43.start
sketch "Spine - long" plane through (0, 0, 0) normal (0, 0, 1) x (1, 0, 0)
  line L0 (-2438.4, 50.8) -> (-2438.4, 101.6)
  line L1 (0, 101.6) -> (0, 50.8)
  line L2 (-2383.8916, 0) -> (-2365.9084, 0) construction
  line L3 (-2365.9084, 0) -> (-2365.9084, 50.8)
  line L4 (-2365.9084, 50.8) -> (-2383.8916, 50.8)
  line L5 (-2383.8916, 50.8) -> (-2383.8916, 0)
  line L6 (-1844.1416, 0) -> (-1826.1584, 0) construction
  line L7 (-1826.1584, 0) -> (-1826.1584, 50.8)
  line L8 (-1826.1584, 50.8) -> (-1844.1416, 50.8)
  line L9 (-1844.1416, 50.8) -> (-1844.1416, 0)
  line L10 (-1304.3916, 0) -> (-1286.4084, 0) construction
  line L11 (-1286.4084, 0) -> (-1286.4084, 50.8)
  line L12 (-1286.4084, 50.8) -> (-1304.3916, 50.8)
  line L13 (-1304.3916, 50.8) -> (-1304.3916, 0)
  line L14 (-764.6416, 0) -> (-764.6416, 50.8)
  line L15 (-764.6416, 50.8) -> (-746.6584, 50.8)
  line L16 (-746.6584, 50.8) -> (-746.6584, 0)
  line L17 (-73.5584, 0) -> (-91.5416, 0)
  line L18 (-91.5416, 0) -> (-91.5416, 50.8)
  line L19 (-91.5416, 50.8) -> (-73.5584, 50.8)
  line L20 (-73.5584, 50.8) -> (-73.5584, 0)
  line L21 (-256.6416, 0) -> (-256.6416, 50.8)
  line L22 (-256.6416, 50.8) -> (-238.6584, 50.8)
  line L23 (-238.6584, 50.8) -> (-238.6584, 0)
  circle A0 centre (-2383.8916, 47.625) radius 3.175
  circle A1 centre (-2365.9084, 47.625) radius 3.175
  circle A2 centre (-256.6416, 47.625) radius 3.175
  circle A3 centre (-238.6584, 47.625) radius 3.175
  circle A4 centre (-91.5416, 47.625) radius 3.175
  circle A5 centre (-73.5584, 47.625) radius 3.175
  line L24 (-73.5584, 50.8) -> (-73.5584, 101.6)
  line L25 (-91.5416, 50.8) -> (-91.5416, 101.6)
  line L26 (-238.6584, 50.8) -> (-238.6584, 101.6)
  line L27 (-256.6416, 50.8) -> (-256.6416, 101.6)
  line L28 (-256.6416, 44.45) -> (-238.6584, 44.45)
  line L29 (-91.5416, 44.45) -> (-73.5584, 44.45)
  circle A6 centre (-1844.1416, 47.625) radius 3.175
  circle A7 centre (-1826.1584, 47.625) radius 3.175
  circle A8 centre (-1304.3916, 47.625) radius 3.175
  circle A9 centre (-1286.4084, 47.625) radius 3.175
  circle A10 centre (-746.6584, 47.625) radius 3.175
  circle A11 centre (-764.6416, 47.625) radius 3.175
  arc A12 (-2438.4, 50.8) -> (-2387.6, 0) centre (-2387.6, 50.8) ccw
  arc A13 (-50.8, 0) -> (0, 50.8) centre (-50.8, 50.8) ccw
  line L30 (-2383.8916, 0) -> (-2387.6, 0)
  line L31 (-1844.1416, 0) -> (-2365.9084, 0)
  line L32 (-1304.3916, 0) -> (-1826.1584, 0)
  line L33 (-764.6416, 0) -> (-1286.4084, 0)
  line L34 (-256.6416, 0) -> (-746.6584, 0)
  line L35 (-746.6584, 0) -> (-764.6416, 0) construction
  line L36 (-50.8, 0) -> (-73.5584, 0)
  line L37 (-238.6584, 0) -> (-256.6416, 0)
  line L38 (-91.5416, 0) -> (-238.6584, 0)
  line L39 (-2438.4, 101.6) -> (-256.6416, 101.6)
  line L40 (-256.6416, 101.6) -> (-238.6584, 101.6)
  line L41 (0, 0) -> (0, 7.62)
  line L42 (0, 7.62) -> (0, 0)
  line L43 (0, 0) -> (-7.62, 0)
  line L44 (-238.6584, 101.6) -> (-91.5416, 101.6)
  line L45 (-73.5584, 101.6) -> (0, 101.6)
  line L46 (-91.5416, 101.6) -> (-73.5584, 101.6)
  point P0 (-2438.4, 0)
  point P1 (-1295.4, 0)
  point P2 (-1835.15, 0)
  point P3 (-2374.9, 0)
  point P4 (-82.55, 0)
  point P5 (-247.65, 0)
  point P6 (-755.65, 0)
  dimension "d834" = 101.6
  dimension "d839" = 17.9832
  dimension "d840" = 50.8
  dimension "d841" = 17.9832
  dimension "d842" = 50.8
  dimension "d843" = 50.8
  dimension "d844" = 17.9832
  dimension "d845" = 539.75
  dimension "d846" = 539.75
  dimension "d847" = 63.5
  dimension "d848" = 17.9832
  dimension "d849" = 50.8
  dimension "d850" = 17.9832
  dimension "d851" = 50.8
  dimension "d852" = 50.8
  dimension "d853" = 17.9832
  dimension "d854" = 539.75
  dimension "d856" = 165.1
  dimension "d857" = 6.35
  dimension "d858" = 6.35
  dimension "d859" = 6.35
  dimension "d860" = 6.35
  dimension "d861" = 6.35
  dimension "d862" = 6.35
  dimension "d863" = 6.35
  dimension "d864" = 6.35
  dimension "d865" = 6.35
  dimension "d866" = 6.35
  dimension "d867" = 6.35
  dimension "d868" = 6.35
  dimension "d984" = 50.8
  dimension "d985" = 50.8
  dimension "d986" = 508
  dimension "d3378" = 2438.4
  dimension "d3379" = 73.8124
  measures "d834" distance of L41.start L1.start
  measures "d839" distance of L2.start L2.end
  measures "d840" distance of L2.start L4.end
  measures "d841" distance of L6.start L6.end
  measures "d842" distance of L6.start L8.end
  measures "d843" distance of L10.start L12.end
  measures "d844" distance of L10.start L10.end
  measures "d845" distance of P1 P2
  measures "d846" distance of P2 P3
  measures "d847" distance of P0 P3
  measures "d848" distance of L16.end L14.start
  measures "d849" distance of L16.end L15.end
  measures "d850" distance of L17.start L17.end
  measures "d851" distance of L17.start L19.end
  measures "d852" distance of L23.end L22.end
  measures "d853" distance of L23.end L21.start
  measures "d854" distance of P1 P6
  measures "d856" distance of P4 P5
  measures "d857" diameter of A0
  measures "d858" diameter of A1
  measures "d859" diameter of A3
  measures "d860" diameter of A2
  measures "d861" diameter of A5
  measures "d862" diameter of A4
  measures "d863" diameter of A7
  measures "d864" diameter of A6
  measures "d865" diameter of A9
  measures "d866" diameter of A8
  measures "d867" diameter of A11
  measures "d868" diameter of A10
  measures "d984" radius of A12
  measures "d985" radius of A13
  measures "d986" distance of P5 P6
  measures "d3378" distance of L0 L1
sketch "Surface" plane through (0, 0, 0) normal (0, 1, 0) x (-1, 0, 0)
  line L0 (0, 0) -> (0, -762)
  line L1 (0, -762) -> (-1828.8, -762)
  line L2 (-1905, -685.8) -> (-1905, 0)
  line L3 (-1905, 0) -> (0, 0)
  arc A0 (-1905, -685.8) -> (-1828.8, -762) centre (-1828.8, -685.8) ccw
  line L4 (-1818.259, -762) -> (-1818.259, 0)
  line L5 (-1828.8, -762) -> (-1828.8, 0) construction
  line L6 (-1839.341, -762) -> (-1839.341, 0)
  line L7 (-1299.591, -762) -> (-1299.591, 0)
  line L8 (-1289.05, -762) -> (-1289.05, 0) construction
  line L9 (-1278.509, -762) -> (-1278.509, 0)
  line L10 (-759.841, -762) -> (-759.841, 0)
  line L11 (-749.3, -762) -> (-749.3, 0) construction
  line L12 (-738.759, -762) -> (-738.759, 0)
  line L13 (-220.091, -762) -> (-220.091, 0)
  line L14 (-209.55, -762) -> (-209.55, 0) construction
  line L15 (-199.009, -762) -> (-199.009, 0)
  dimension "d3039" = 1905
  dimension "d3040" = 762
  dimension "d3041" = 76.2
  dimension "d3042" = 10.541
  dimension "d3043" = 10.541
  dimension "d3045" = 10.541
  dimension "d3046" = 10.541
  dimension "d3047" = 539.75
  dimension "d3048" = 10.541
  dimension "d3049" = 10.541
  dimension "d3050" = 10.541
  dimension "d3051" = 10.541
  dimension "d3052" = 539.75
  dimension "d3053" = 539.75
  dimension "d3377" = 76.2
  measures "d3039" distance of L2.end L0.start
  measures "d3040" distance of L0.start L0.end
  measures "d3041" radius of A0
  measures "d3042" distance of L4 L5
  measures "d3043" distance of L5 L6
  measures "d3045" distance of L7 L8
  measures "d3046" distance of L8 L9
  measures "d3047" distance of L5 L8
  measures "d3048" distance of L10 L11
  measures "d3049" distance of L11 L12
  measures "d3050" distance of L13 L14
  measures "d3051" distance of L14 L15
  measures "d3052" distance of L8 L11
  measures "d3053" distance of L11 L14
  measures "d3377" distance of L2 L5
extrude "Extrude1" add sketch "Inner end leg" along normal blind 18.542 contours A0 L1 L2 L3 A1 L4 A2 A3 A4 A5 L6 L7 L8 L9 A6 A7 L10 L12 A8 L14 A9 L15 L17 L19 L20 L21 L22 A18 L31 L32 L33 L34 L35 L36 L38 L39 L40 L42 A19 A20 makes body 1 in component "Inner leg end"
extrude "Extrude1'" add sketch "Inner leg" along normal blind 18.542 separate body contours L0 L1 L2 A0 A1 L4 L5 A2 L6 A3 L7 L9 L10 L12 A4 A5 L13 L14 L16 A6 A7 L18 L19 L20 L22 L23 L24 A8 A9 A10 A11 L34 L35 L36 L37 L38 L39 L40 A23 A24 L43 L44 L45 A25 makes body 2 in component "Inner leg - left -- right"
extrude "Extrude1''" add sketch "Inner leg" along normal blind 18.542 separate body contours L0 L1 L2 A0 A1 L4 L5 A2 L6 A3 L7 L9 L10 L12 A4 A5 L13 L14 L16 A6 A7 L18 L19 L20 L22 L23 L24 A8 A9 A10 A11 L34 L35 L36 L37 L38 L39 L40 A23 A24 L43 L44 L45 A25 makes body 3 in component "Inner leg - right -- right"
extrude "Extrude1'''" add sketch "Inner leg" along normal blind 18.542 separate body contours L0 L1 L2 A0 A1 L4 L5 A2 L6 A3 L7 L9 L10 L12 A4 A5 L13 L14 L16 A6 A7 L18 L19 L20 L22 L23 L24 A8 A9 A10 A11 L34 L35 L36 L37 L38 L39 L40 A23 A24 L43 L44 L45 A25 makes body 4 in component "Inner leg - right -- middle"
extrude "Extrude1''''" add sketch "Inner leg" along normal blind 18.542 separate body contours L0 L1 L2 A0 A1 L4 L5 A2 L6 A3 L7 L9 L10 L12 A4 A5 L13 L14 L16 A6 A7 L18 L19 L20 L22 L23 L24 A8 A9 A10 A11 L34 L35 L36 L37 L38 L39 L40 A23 A24 L43 L44 L45 A25 makes body 5 in component "Inner leg - right -- left"
extrude "Extrude1'''''" add sketch "Inner leg" along normal blind 18.542 separate body contours L0 L1 L2 A0 A1 L4 L5 A2 L6 A3 L7 L9 L10 L12 A4 A5 L13 L14 L16 A6 A7 L18 L19 L20 L22 L23 L24 A8 A9 A10 A11 L34 L35 L36 L37 L38 L39 L40 A23 A24 L43 L44 L45 A25 makes body 6 in component "Inner leg - left -- left"
extrude "Extrude1''''''" add sketch "Spine - long" along normal blind 18.542 separate body contours L0 L3 L4 L5 L7 L8 L9 L11 L12 L13 L14 L15 L16 L21 A0 A1 A2 L27 A6 A7 A8 A9 A10 A11 A12 L30 L31 L32 L33 L34 L39 | L22 L26 L27 L40 | L18 L23 A3 A4 L25 L26 L38 L44 | L19 L24 L25 L46 | L1 L20 A5 L24 A13 L36 L45 | L20 A5 picked at (-72.5108, 47.7756) makes body 7 in component "Long spine (1)"
extrude "Extrude1'''''''" add sketch "Spine - short" along normal blind 18.542 separate body contours L0 L1 L3 L4 L5 L6 L7 L8 L10 L11 L12 L14 L15 L16 A0 A1 A2 A3 A4 A5 A6 A7 L17 L18 L19 L20 L21 L22 A8 A9 A10 A11 A12 A13 L23 L24 L26 L27 L29 L30 L32 L33 makes body 8 in component "Short spine"
extrude "Extrude1''''''''" add sketch "End leg - wave" along normal blind 18.542 separate body contours A0 A2 L0 L1 L2 L3 A4 L5 L6 L7 A5 A6 A7 L8 L13 L22 A21 A23 L30 L41 L42 L43 A32 | A3 A9 L22 A21 | A1 A3 A8 L10 L12 L16 L20 A9 L22 L23 L24 L25 L26 L27 A11 A13 A15 A17 L33 L34 L35 L36 L37 L38 L39 L40 A33 makes body 9 in component "End leg - right (1)"
extrude "Extrude2" cut sketch "End leg - wave" along normal blind 2.54 contours A3 A9 L22 A21 bodies 9 in component "End leg - right (1)"
extrude "Extrude1'''''''''" add sketch "End leg - wave" against normal blind 18.542 separate body contours A0 A2 L0 L1 L2 L3 A4 L5 L6 L7 A5 A6 A7 L8 L13 L22 A21 A23 L30 L41 L42 L43 A32 | A3 A9 L22 A21 | A1 A3 A8 L10 L12 L16 L20 A9 L22 L23 L24 L25 L26 L27 A11 A13 A15 A17 L33 L34 L35 L36 L37 L38 L39 L40 A33 makes body 10 in component "End leg - left (1)"
extrude "Extrude2'" cut sketch "End leg - wave" against normal blind 2.54 contours A3 A9 L22 A21 bodies 10 in component "End leg - left (1)"
extrude "Extrude1''''''''''" add sketch "Surface" along normal blind 18.542 separate body makes body 11 in component "Surface - left"
extrude "Extrude2''" cut sketch "Surface" along normal blind 6.1807 contours L1 L3 L13 L15 | L1 L3 L10 L12 | L1 L3 L7 L9 | L1 L3 A0 L4 L6 bodies 11 in component "Surface - left"
extrude "Extrude1'''''''''''" add sketch "Surface" against normal blind 18.542 separate body makes body 12 in component "Surface - right"
extrude "Extrude2'''" cut sketch "Surface" against normal blind 6.1807 contours L1 L3 L13 L15 | L1 L3 L10 L12 | L1 L3 L7 L9 | L1 L3 A0 L4 L6 bodies 12 in component "Surface - right"
extrude "Extrude1''''''''''''" add sketch "Shelf" along normal blind 18.542 separate body contours L0 L1 L2 L3 L4 L5 A0 A1 A2 A3 L8 L9 L10 L12 L13 L14 L15 L16 L17 A4 A5 A6 A7 A8 A9 A10 A11 L18 L19 L20 L22 L23 makes body 13 in component "Shelf - right -- upper"
extrude "Extrude1'''''''''''''" add sketch "Shelf" along normal blind 18.542 separate body contours L0 L1 L2 L3 L4 L5 A0 A1 A2 A3 L8 L9 L10 L12 L13 L14 L15 L16 L17 A4 A5 A6 A7 A8 A9 A10 A11 L18 L19 L20 L22 L23 makes body 14 in component "Shelf - right -- lower"
extrude "Extrude1''''''''''''''" add sketch "Shelf" along normal blind 18.542 separate body contours L0 L1 L2 L3 L4 L5 A0 A1 A2 A3 L8 L9 L10 L12 L13 L14 L15 L16 L17 A4 A5 A6 A7 A8 A9 A10 A11 L18 L19 L20 L22 L23 makes body 15 in component "Shelf - left -- upper"
copy_body "CopyPasteBodies1" bodies 15 makes body 16 in component "Shelf - left -- lower"
sketch "4x8' sheet" plane through (0, 0, 0) normal (0, 1, 0) x (1, 0, 0)
  line L0 (0, 0) -> (2438.4, 0)
  line L1 (2438.4, 0) -> (2438.4, -1219.2)
  line L2 (2438.4, -1219.2) -> (0, -1219.2)
  line L3 (0, -1219.2) -> (0, 0)
  dimension "d3594" = 2438.4
  dimension "d3596" = 1219.2
  measures "d3594" distance of L0.start L0.end
  measures "d3596" distance of L0.end L1.end
extrude "Extrude1'''''''''''''''" add sketch "4x8' sheet" along normal blind 18.542 separate body makes body 17 in component "Stock - 4x8'"
sketch "4x4' sheet" plane through (0, 0, 0) normal (0, 1, 0) x (1, 0, 0)
  line L0 (0, 0) -> (1219.2, 0)
  line L1 (1219.2, 0) -> (1219.2, -1219.2)
  line L2 (1219.2, -1219.2) -> (0, -1219.2)
  line L3 (0, -1219.2) -> (0, 0)
  dimension "d3597" = 1219.2
  dimension "d3598" = 1219.2
  measures "d3597" distance of L0.start L0.end
  measures "d3598" distance of L0.start L2.end
extrude "Extrude1''''''''''''''''" add sketch "4x4' sheet" along normal blind 18.542 separate body makes body 18 in component "Stock - 4x4'"
extrude "Extrude1'''''''''''''''''" add sketch "End leg - wave" along normal blind 18.542 separate body contours A0 A2 L0 L1 L2 L3 A4 L5 L6 L7 A5 A6 A7 L8 L13 L22 A21 A23 L30 L41 L42 L43 A32 | A3 A9 L22 A21 | A1 A3 A8 L10 L12 L16 L20 A9 L22 L23 L24 L25 L26 L27 A11 A13 A15 A17 L33 L34 L35 L36 L37 L38 L39 L40 A33 makes body 19 in component "End leg - right (1) (1)"
extrude "Extrude2''''" cut sketch "End leg - wave" along normal blind 2.54 contours A3 A9 L22 A21 bodies 19 in component "End leg - right (1) (1)"
extrude "Extrude1''''''''''''''''''" add sketch "Inner leg" along normal blind 18.542 separate body contours L0 L1 L2 A0 A1 L4 L5 A2 L6 A3 L7 L9 L10 L12 A4 A5 L13 L14 L16 A6 A7 L18 L19 L20 L22 L23 L24 A8 A9 A10 A11 L34 L35 L36 L37 L38 L39 L40 A23 A24 L43 L44 L45 A25 makes body 20 in component "Inner leg - right -- right (1)"
extrude "Extrude1'''''''''''''''''''" add sketch "End leg - wave" against normal blind 18.542 separate body contours A0 A2 L0 L1 L2 L3 A4 L5 L6 L7 A5 A6 A7 L8 L13 L22 A21 A23 L30 L41 L42 L43 A32 | A3 A9 L22 A21 | A1 A3 A8 L10 L12 L16 L20 A9 L22 L23 L24 L25 L26 L27 A11 A13 A15 A17 L33 L34 L35 L36 L37 L38 L39 L40 A33 makes body 21 in component "End leg - left (1) (1)"